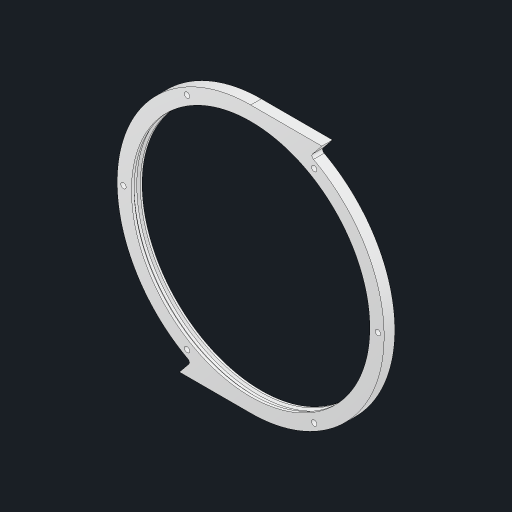
# Autodesk Inventor part: Weapon Disk One Part
Saved by Autodesk Inventor 2023.2 (Build 272271030, 271C)
## iProperties
Created: 2024-02-21
Part Number: Weapon Disk One Part
Material: Aluminum 6061
Document SubType Name: Modeling
Designer: robpl
Density: 2.7 g/cm^3
Appearance: Aluminum - Flat
Mass: 57.9341 g
Surface Area: 137.369 cm^2
Volume: 21.4571 cm^3
Author: robpl
Autodesk Inventor part; units mm, degrees
ref_plane "YZ Plane" through (0, 0, 0) normal (1, 0, 0) x (0, 1, 0)
ref_plane "XZ Plane" through (0, 0, 0) normal (0, 1, 0) x (-1, 0, 0)
ref_plane "XY Plane" through (0, 0, 0) normal (0, 0, 1) x (1, 0, 0)
sketch "Sketch1" plane through (0, 0, 0) normal (0, 0, 1) x (1, 0, 0)
  circle A0 centre (0, 0) radius 67
  circle A1 centre (0, 0) radius 75
  line L0 (0, 75) -> (40, 75)
  line L1 (40, 75) -> (0, 0)
  line L2 (40, 75) -> (33.5659, 67.0696)
  arc A2 (34.8046, 68.5963) -> (35.2941, 66.1765) centre (36.0471, 67.5882) ccw
  line L3 (0, 0) -> (23.5794, 0)
  line L4 (0, -75) -> (-40, -75)
  line L5 (-40, -75) -> (-33.5659, -67.0696)
  arc A3 (-34.8046, -68.5963) -> (-35.2941, -66.1765) centre (-36.0471, -67.5882) ccw
  line L6 (0, 0) -> (0, 17.5372)
  point P0 (-35.2941, -66.1765)
  dimension "d0" = 134
  dimension "d1" = 150
  dimension "d2" = 10
  dimension "d3" = 1.6
  dimension "d6" = 360
  constraints: 14 end point, 7 point on circle, 4 centre point, 3 point on line, 2 coincident, 2 horizontal, 2 tangent, 1 vertical, 1 vertical alignment, 19 other
  measures "d0" diameter of A0
  measures "d1" diameter of A1
  measures "d2" distance of L0.end A2.end
  measures "d3" radius of A2
extrude "Extrusion1" add sketch "Sketch1" along normal blind 6 contours A1
extrude "Extrusion2" add sketch "Sketch1" along normal blind 6 contours A1 L2 A2 | A1 L0 L2
sketch "Sketch4" plane through (0, 0, 0) normal (1, 0, 0) x (0, 1, 0)
  line L0 (67, 6) -> (67, 0) projected
  line L1 (67, 4.5) -> (68, 3.5)
  line L2 (68, 3.5) -> (68, 2)
  line L3 (68, 2) -> (67, 1)
  line L4 (61.5, 4) -> (61.5, 1.5)
  line L5 (61.5, 1.5) -> (67.5, 1.5)
  line L6 (67.5, 1.5) -> (67.5, 4)
  line L7 (67.5, 4) -> (61.5, 4)
  line L8 (-13.6, 0) -> (81.6, 0) projected
  line L9 (0, -1.2) -> (0, 7.2) projected
  point P0 (0, 0)
  dimension "d24" = 6
  dimension "d25" = 2.5
  dimension "d27" = 1
  dimension "d28" = 0.5
  dimension "d29" = 0.5
  constraints: 14 end point, 5 perpendicular, 2 midpoint, 2 parallel, 2 point on line
  measures "d24" distance of L5.end L4.end
  measures "d25" distance of L4.end L4.start
  measures "d27" distance of L0.end L3.end
  measures "d28" distance between parallel lines of L2 L6
  measures "d29" distance between parallel lines of L0 L6
revolve "Revolution1" cut sketch "Sketch4" angle 360 about axis through (0, 0, -10) along (0, 0, 1) contours L1 L7 L0 | L7 L6 L5 L0 | L1 L2 L3 L6 | L5 L3 L0
sketch "Sketch2" plane through (0, 0, 6) normal (0, 0, 1) x (1, 0, 0)
  circle A0 centre (71.5, 0) radius 1.5
  arc A1 (0, 75) -> (35.2941, 66.1765) centre (0, 0) ccw projected
  circle A2 centre (0, 0) radius 75
  circle A3 centre (71.5, 0) radius 3.5
  circle A4 centre (0, 0) radius 68 projected
  point P0 (26.0989, -70.3125)
  dimension "d12" = 3
  constraints: 3 centre point, 2 coincident, 2 tangent, 1 horizontal alignment, 1 point on circle
  measures "d12" diameter of A0
extrude "Extrusion3" cut sketch "Sketch2" against normal through all contours A0
sketch "Sketch3" plane through (0, 0, 6) normal (0, 0, 1) x (1, 0, 0)
  circle A0 centre (71.5, 0) radius 1.5 projected
  circle A1 centre (71.5, 0) radius 75
  line L0 (-27.8388, 75) -> (40, 75) projected
  circle A2 centre (71.5, 0) radius 99.3657
  point P0 (0, 0)
  point P1 (-0.97, 69.9933)
  point P2 (0.97, 69.9933)
  point P3 (-0.97, 69.9933)
  constraints: 2 coincident, 1 centre point, 1 tangent, 4 other
extrude "Extrusion4" [suppressed]
fillet "Fillet1" [suppressed]
pattern_circular "Circular Pattern1" count 6 over 360 about axis through (0, 0, 0) along (0, 0, 1) of "Extrusion3"
pattern_circular "Circular Pattern2" count 2 over 360 about axis through (0, 0, 0) along (0, 0, 1) of "Extrusion2"
body "Solid1"
